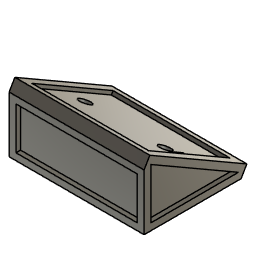
WaterHolder (Autodesk Fusion 360 design; units mm, degrees)
Autodesk Fusion 360 part; units mm, degrees
sketch "Sketch1" plane through (0, 0, 0) normal (0, 0, 1) x (1, 0, 0)
  line L0 (-38, 18.4) -> (162, 18.4)
  line L1 (162, 18.4) -> (162, -131.6)
  line L2 (162, -131.6) -> (-38, -131.6)
  line L3 (-38, -131.6) -> (-38, 18.4)
  dimension "d1" = 200
  dimension "d2" = 150
  constraint horizontal L0
  constraint vertical L1
  constraint horizontal L2
  constraint vertical L3
  measures "d1" distance of L0.start L0.end
  measures "d2" distance of L0.start L2.end
extrude "Extrude1" add sketch "Sketch1" along normal blind 5 makes body 1
sketch "Sketch2" plane through (0, 0, 5) normal (0, 0, 1) x (-1, 0, 0)
  line L0 (38, 131.6) -> (-162, 131.6)
  line L1 (-162, 131.6) -> (-162, -18.4)
  line L2 (-162, -18.4) -> (38, -18.4)
  line L3 (38, -18.4) -> (38, 131.6)
  line L4 (-30.8, 31.6) -> (-85.8, 31.6)
  line L5 (-85.8, 31.6) -> (-85.8, 76.6)
  line L6 (-85.8, 76.6) -> (-30.8, 76.6)
  line L7 (-30.8, 76.6) -> (-30.8, 31.6)
  dimension "d5" = 55
  dimension "d6" = 45
  constraint horizontal L4
  constraint vertical L5
  constraint horizontal L6
  constraint vertical L7
  measures "d5" distance of L4.start L4.end
  measures "d6" distance of L4.start L6.end
extrude "Extrude2" add sketch "Sketch2" along normal blind 5 separate body contours L4 L5 L6 L7 makes body 2
move_body "Move1" bodies 2 to x (0.866025, 0, 0.5) y (0, 1, 0) z (-0.5, 0, 0.866025) at (5.3107, 0, -14.8199)
move_body "Move2" bodies 2 to x (0.866025, 0, -0.5) y (0, 1, 0) z (0.5, 0, 0.866025) at (-12.8736, 0, 50.0244)
extrude "Extrude3" add 1 faces at (51.7824, -76.6, 41.2013) along direction (0, -1, 0) blind 2 on bodies 2 bodies 2
extrude "Extrude4" add 1 faces at (15.1157, -62.9333, 41.2013) along direction (-1, 0, 0) blind 2 on bodies 2 bodies 2
extrude "Extrude5" add 1 faces at (32.1157, -31.6, 41.2013) along direction (0, 1, 0) blind 2 on bodies 2 bodies 2
extrude "Extrude6" add 1 faces at (70.1157, -62.2667, 41.2013) along direction (1, 0, 0) blind 2 on bodies 2 bodies 2
sketch "Sketch4" plane through (0, 0, 44.5346) normal (0, 0, 1) x (-1, 0, 0)
  line L0 (-72.1157, 29.6) -> (-13.1157, 29.6)
  line L1 (-13.1157, 29.6) -> (-13.1157, 78.6)
  line L2 (-13.1157, 78.6) -> (-72.1157, 78.6)
  line L3 (-72.1157, 78.6) -> (-72.1157, 29.6)
  line L4 (-68.1157, 74.6) -> (-17.1157, 74.6)
  line L5 (-17.1157, 74.6) -> (-17.1157, 33.6)
  line L6 (-17.1157, 33.6) -> (-68.1157, 33.6)
  line L7 (-68.1157, 33.6) -> (-68.1157, 74.6)
  dimension "d19" = 51
  dimension "d20" = 41
  dimension "d21" = 4
  dimension "d22" = 4
  constraint horizontal L4
  constraint vertical L5
  constraint horizontal L6
  constraint vertical L7
  measures "d19" distance of L4.start L4.end
  measures "d20" distance of L4.start L6.end
  measures "d21" distance of L3 L7
  measures "d22" distance of L2 L4
extrude "Extrude7" cut sketch "Sketch4" against normal blind 1.5 contours L4 L5 L6 L7 bodies 2
move_body "Move3" bodies 2 to x (1, 0, 0) y (0, 0.866025, -0.5) z (0, 0.5, 0.866025) at (0, -28.7653, -21.2845)
sketch "Sketch5" plane through (13.1157, 0, 0) normal (-1, 0, 0) x (0, -1, 0)
  line L0 (34.6324, 27.7535) -> (77.0676, 52.2535)
  line L1 (77.0676, 52.2535) -> (74.5676, 56.5836)
  line L2 (74.5676, 56.5836) -> (32.1324, 32.0836)
  line L3 (32.1324, 32.0836) -> (34.6324, 27.7535)
  line L4 (34.6324, 27.7535) -> (77.0676, 27.7535)
  line L5 (77.0676, 52.2535) -> (77.0676, 27.7535)
  constraint coincident L0.start L3.end
  constraint horizontal L4
  constraint coincident L0.end L1.start
  constraint coincident L4 L5.end
  constraint perpendicular L4 L5
extrude "Extrude8" add sketch "Sketch5" against normal blind 59 contours L0 L4 L5 bodies 2
sketch "Sketch6" plane through (13.1157, 0, 0) normal (-1, 0, 0) x (0, -1, 0)
  line L0 (77.0676, 52.2535) -> (74.5676, 56.5836)
  line L1 (74.5676, 56.5836) -> (32.1324, 32.0836)
  line L2 (32.1324, 32.0836) -> (34.6324, 27.7535)
  line L3 (34.6324, 27.7535) -> (77.0676, 27.7535)
  line L4 (77.0676, 27.7535) -> (77.0676, 52.2535)
  line L5 (74.0676, 30.7535) -> (74.0676, 52.8309)
  line L6 (74.0676, 52.8309) -> (35.8285, 30.7535)
  line L7 (74.0676, 30.7535) -> (70.6676, 30.7535)
  line L8 (70.6676, 30.7535) -> (35.8285, 30.7535)
  dimension "d28" = 60
  dimension "d29" = 3
  dimension "d30" = 3
  dimension "d31" = 3
  constraint vertical L5
  constraint perpendicular L5 L7
  constraint perpendicular L5 L8
  constraint coincident L6.end L8
  measures "d28" angle of L5 L6
  measures "d29" distance of L1 L6
  measures "d30" distance of L4 L5
  measures "d31" distance of L3 L8
extrude "Extrude9" cut sketch "Sketch6" against normal blind 2 contours L5 L6 L7 L8 bodies 2
sketch "Sketch8" plane through (72.1157, 0, 0) normal (1, 0, 0) x (0, 1, 0)
  line L0 (-34.6324, 27.7535) -> (-32.1324, 32.0836)
  line L1 (-32.1324, 32.0836) -> (-74.5676, 56.5836)
  line L2 (-74.5676, 56.5836) -> (-77.0676, 52.2535)
  line L3 (-77.0676, 52.2535) -> (-77.0676, 27.7535)
  line L4 (-77.0676, 27.7535) -> (-34.6324, 27.7535)
  line L5 (-74.0676, 52.8309) -> (-74.0676, 30.7535)
  line L6 (-74.0676, 52.8309) -> (-35.7761, 30.7233)
  line L7 (-74.0676, 52.8309) -> (-44.3867, 52.8309) construction
  line L8 (-74.0676, 30.7535) -> (-35.8, 30.7535)
  dimension "d38" = 30
  dimension "d39" = 3
  dimension "d40" = 3
  dimension "d41" = 3
  constraint vertical L5
  constraint horizontal L7
  constraint perpendicular L5 L8
  measures "d38" angle of L6 L7
  measures "d39" distance of L1 L6
  measures "d40" distance of L3 L5
  measures "d41" distance of L4 L8
extrude "Extrude10" cut sketch "Sketch8" against normal blind 2 contours L5 L6 L8 bodies 2
sketch "Sketch9" plane through (0, -77.0676, 0) normal (0, -1, 0) x (1, 0, 0)
  line L0 (13.1157, 52.2535) -> (13.1157, 27.7535)
  line L1 (13.1157, 27.7535) -> (72.1157, 27.7535)
  line L2 (72.1157, 27.7535) -> (72.1157, 52.2535)
  line L3 (72.1157, 52.2535) -> (13.1157, 52.2535)
  line L4 (16.1157, 49.2535) -> (69.1157, 49.2535)
  line L5 (69.1157, 49.2535) -> (69.1157, 30.7535)
  line L6 (69.1157, 30.7535) -> (16.1157, 30.7535)
  line L7 (16.1157, 30.7535) -> (16.1157, 49.2535)
  dimension "d44" = 3
  dimension "d45" = 3
  dimension "d46" = 3
  dimension "d47" = 3
  constraint horizontal L4
  constraint vertical L5
  constraint horizontal L6
  constraint vertical L7
  measures "d44" distance of L3 L4
  measures "d45" distance of L0 L7
  measures "d46" distance of L2 L5
  measures "d47" distance of L1 L6
extrude "Extrude11" cut sketch "Sketch9" against normal blind 2 contours L4 L5 L6 L7 bodies 2
sketch "Sketch10" plane through (0, 5.1095, 8.85) normal (0, 0.5, 0.866025) x (-1, 0, 0)
  line L0 (-68.1157, 47.8693) -> (-17.1157, 47.8693)
  line L1 (-17.1157, 47.8693) -> (-17.1157, 88.8693)
  line L2 (-17.1157, 88.8693) -> (-68.1157, 88.8693)
  line L3 (-68.1157, 88.8693) -> (-68.1157, 47.8693)
  line L4 (-66.1157, 71.8693) -> (-63.1157, 71.8693)
  line L5 (-63.1157, 71.8693) -> (-63.1157, 64.8693)
  line L6 (-63.1157, 64.8693) -> (-66.1157, 64.8693)
  line L7 (-66.1157, 64.8693) -> (-66.1157, 71.8693)
  dimension "d50" = 3
  dimension "d51" = 7
  dimension "d52" = 17
  dimension "d53" = 2
  constraint horizontal L4
  constraint vertical L5
  constraint horizontal L6
  constraint vertical L7
  measures "d50" distance of L4.start L4.end
  measures "d51" distance of L4.start L6.end
  measures "d52" distance of L2 L4
  measures "d53" distance of L3 L7
extrude "Extrude12" cut sketch "Sketch10" against normal blind 32 contours L4 L5 L6 L7 bodies 2
sketch "Sketch11" plane through (0, 0, 27.7535) normal (0, 0, -1) x (1, 0, 0)
  line L0 (63.1157, 58.8811) -> (63.1157, 66.964)
  line L1 (63.1157, 66.964) -> (66.1157, 66.964)
  line L2 (66.1157, 66.964) -> (66.1157, 58.8811)
  line L3 (66.1157, 58.8811) -> (63.1157, 58.8811)
  line L4 (13.1157, 77.0676) -> (13.1157, 34.6324)
  line L5 (13.1157, 34.6324) -> (72.1157, 34.6324)
  line L6 (72.1157, 34.6324) -> (72.1157, 77.0676)
  line L7 (72.1157, 77.0676) -> (13.1157, 77.0676)
  circle A0 centre (25.1157, 55.8424) radius 1.5
  circle A1 centre (60.1157, 55.8424) radius 1.5
  line L8 (13.1157, 35.8285) -> (13.1157, 74.0676)
  line L9 (72.1157, 32.1324) -> (72.1157, 74.5676)
  dimension "d56" = 3
  dimension "d57" = 3
  dimension "d58" = 12
  dimension "d59" = 12
  dimension "d60" = 21.21
  dimension "d61" = 21.21
  measures "d56" diameter of A0
  measures "d57" diameter of A1
  measures "d58" distance of A0.centre L8
  measures "d59" distance of A1.centre L9
  measures "d60" distance of L5 A0.centre
  measures "d61" distance of L5 A1.centre
extrude "Extrude13" cut sketch "Sketch11" against normal blind 24 contours A0 | A1 bodies 2
sketch "Sketch12" plane through (0, 0, 27.7535) normal (0, 0, -1) x (1, 0, 0)
  circle A0 centre (25.1157, 55.8424) radius 1.5
  circle A1 centre (60.1157, 55.8424) radius 1.5
  line L0 (63.1157, 58.8811) -> (63.1157, 66.964)
  line L1 (63.1157, 66.964) -> (66.1157, 66.964)
  line L2 (66.1157, 66.964) -> (66.1157, 58.8811)
  line L3 (66.1157, 58.8811) -> (63.1157, 58.8811)
  line L4 (13.1157, 77.0676) -> (13.1157, 34.6324)
  line L5 (13.1157, 34.6324) -> (72.1157, 34.6324)
  line L6 (72.1157, 34.6324) -> (72.1157, 77.0676)
  line L7 (72.1157, 77.0676) -> (13.1157, 77.0676)
  circle A2 through (62.6157, 55.8424, -20) (58.8657, 58.0074, -20) (58.8657, 53.6773, -20)
  circle A3 through (27.6157, 55.8424, -20) (23.8657, 58.0074, -20) (23.8657, 53.6773, -20)
  dimension "d64" = 5
  dimension "d65" = 5
extrude "Extrude14" cut sketch "Sketch12" along normal blind 17 contours A2 | A3 in plane through (0, 0, 47.7535) normal (0, 0, -1) bodies 2
hidden bodies 1
